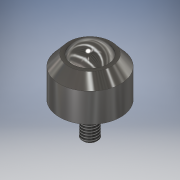
# Autodesk Inventor part: ball_unit_11mi-16-13_reformed
Saved by Autodesk Inventor 2019 (Build 230136000, 136)
## iProperties
Created: 2021-03-26
Part Number: ball_unit_11mi-16-13_reformed
Material: Steel, High Strength, Low Alloy
Document SubType Name: Modeling
Designer: rtavi
Density: 7.85 g/cm^3
Appearance: Steel - Polished
Mass: 58.0341 g
Surface Area: 25.6912 cm^2
Volume: 7.39288 cm^3
Author: rtavi
Autodesk Inventor part; units mm, degrees
ref_plane "YZ Plane" through (0, 0, 0) normal (1, 0, 0) x (0, 1, 0)
ref_plane "XZ Plane" through (0, 0, 0) normal (0, 1, 0) x (-1, 0, 0)
ref_plane "XY Plane" through (0, 0, 0) normal (0, 0, 1) x (1, 0, 0)
sketch "Sketch1" plane through (0, 0, 0) normal (0, 0, 1) x (1, 0, 0)
  line L0 (0.9, -11) -> (-0.9, -11) construction
  line L1 (-0.9, -11) -> (-0.9, -11.4588) construction
  line L2 (-0.9, -11.4588) -> (-0.9, -12) construction
  line L3 (-0.9, -12) -> (-2.4588, -12) construction
  line L4 (-2.4588, -12) -> (-3, -11.4588)
  line L5 (-3, -11.4588) -> (-3, 0)
  line L6 (8.4, 0) -> (-8.4, 0) construction
  line L7 (-8.4, 0) -> (-9.4, 1)
  line L8 (12, 1) -> (-12, 1) construction
  line L9 (-12, 1) -> (-12, 12.3)
  line L10 (-12, 12.3) -> (-8.4, 16.5)
  line L11 (8.4, 16.5) -> (-8.4, 16.5) construction
  line L12 (8, 12.6) -> (-8, 12.6) construction
  arc A0 (-6.985, 16.5) -> (-8, 12.6) centre (0, 12.6) ccw
  line L13 (-8.4, 16.5) -> (-6.985, 16.5)
  line L14 (0, 20.5) -> (0, -11)
  line L15 (-8, 12.6) -> (-7.9, 12.6)
  line L16 (-12, 1) -> (-9.4, 1)
  line L17 (-8.4, 0) -> (-3, 0)
  line L18 (-2.4588, -12) -> (-0.9, -12)
  line L19 (-0.9, -11) -> (-0.9, -12)
  line L20 (-0.9, -11) -> (0, -11)
  arc A1 (0, 20.5) -> (-7.9, 12.6) centre (0, 12.6) ccw
  point P0 (0, 0)
  constraints: 26 end point, 4 point on circle, 3 perpendicular, 2 centre point, 2 horizontal, 2 vertical, 1 collinear, 1 midpoint, 1 point on line, 14 other
revolve "Revolution1" add sketch "Sketch1" angle 360 about axis through (0, 20.5, 0) along (0, -1, 0)
thread "Thread1" size "M6x1" class "6g" standard "ANSI Metric M Profile" full length
body "Solid1"
